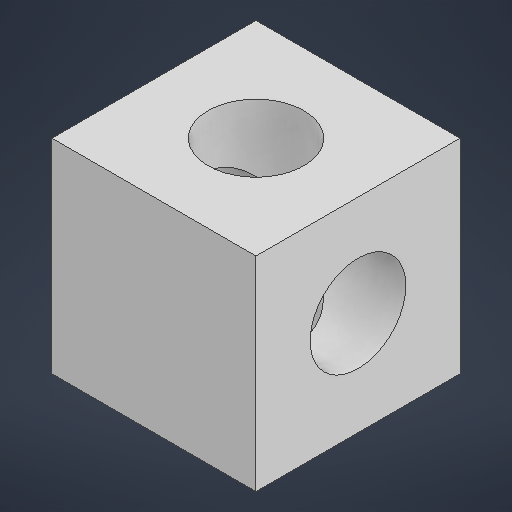
# Autodesk Inventor part: peca3
Saved by Autodesk Inventor 2026.2 (Build 302298000, 298)
## iProperties
Created: 2026-09-25
Part Number: peca3
Material: Genérico
Document SubType Name: Modeling
Designer: IFSP
Density: 1 g/cm^3
Appearance: Padrão
Author: IFSP
Autodesk Inventor part; units mm, degrees
ref_plane "YZ Plane" through (0, 0, 0) normal (1, 0, 0) x (0, 1, 0)
ref_plane "XZ Plane" through (0, 0, 0) normal (0, 1, 0) x (-1, 0, 0)
ref_plane "XY Plane" through (0, 0, 0) normal (0, 0, 1) x (1, 0, 0)
sketch "Esboço1" plane through (0, 0, 0) normal (0, 1, 0) x (-1, 0, 0)
  line L0 (10.16, 10.16) -> (-10.16, 10.16)
  line L1 (-10.16, 10.16) -> (-10.16, -10.16)
  line L2 (-10.16, -10.16) -> (10.16, -10.16)
  line L3 (10.16, -10.16) -> (10.16, 10.16)
  line L4 (10.16, 10.16) -> (-10.16, -10.16) construction
  line L5 (-10.16, 10.16) -> (10.16, -10.16) construction
  line L6 (0, 22.6457) -> (0, -28.8984) construction
  circle A0 centre (0, 0) radius 4.765
  point P0 (0, -10.16)
  dimension "d1" = 20.32
  dimension "d2" = 10.16
  dimension "d3" = 9.53
  constraints: 14 end point, 3 midpoint, 2 parallel, 1 centre point, 1 coincident, 1 horizontal, 1 perpendicular, 1 vertical
  measures "d1" distance of L1.end L0.end
  measures "d2" distance of point (0, -10.16) L1.end
  measures "d3" diameter of A0
extrude "Extrusão1" add sketch "Esboço1" along normal blind 20.32
sketch "Esboço2" plane through (10.16, 0, 10.16) normal (1, 0, 0) x (0, 0, -1)
  line L0 (0, 0) -> (20.32, 0) projected
  line L1 (10.16, 0) -> (0, 0)
  line L2 (10.16, 21.153) -> (10.16, -10.5872) construction
  circle A0 centre (10.16, 10.2866) radius 4.765
  dimension "d6" = 10.16
  dimension "d7" = 9.53
  constraints: 4 end point, 1 centre point, 1 collinear, 1 midpoint, 1 point on line, 1 vertical
  measures "d6" distance of L0.start point (10.16, 0)
  measures "d7" diameter of A0
extrude "Extrusão2" cut sketch "Esboço2" against normal blind 20.32
